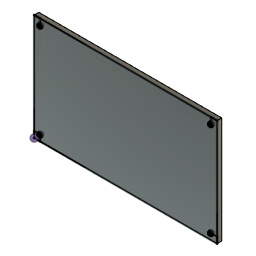
noyce 64 button backing (Autodesk Fusion 360 design; units mm, degrees)
Autodesk Fusion 360 part; units mm, degrees
note: some values were not read from the file. Set by a fixed rule: which sketch regions a step uses.
sketch "Sketch1" plane through (0, 0, 0) normal (0, 1, 0) x (1, 0, 0)
  line L0 (0, 0) -> (79, 0)
  line L1 (79, 0) -> (79, -46)
  line L2 (79, -46) -> (0, -46)
  line L3 (0, -46) -> (0, 0)
  line L4 (79, -46) -> (76.365, -46)
  line L5 (76.365, -46) -> (76.365, -43.365)
  line L6 (79, 0) -> (79, -2.635)
  line L7 (79, -2.635) -> (76.365, -2.635)
  line L8 (0, -46) -> (2.635, -46)
  line L9 (2.635, -46) -> (2.635, -43.365)
  line L10 (0, 0) -> (2.635, 0)
  line L11 (2.635, 0) -> (2.635, -2.635)
  line L12 (2.635, -2.635) -> (0, -2.635)
  line L13 (0, -2.635) -> (0, 0)
  circle A0 centre (76.365, -43.365) radius 0.8
  circle A1 centre (76.365, -2.635) radius 0.8
  circle A2 centre (2.635, -2.635) radius 0.8
  circle A3 centre (2.635, -43.365) radius 0.8
  dimension "d1" = 46
  dimension "d2" = 79
  dimension "d5" = 2.635
  dimension "d6" = 2.635
  dimension "d7" = 2.635
  dimension "d8" = 2.635
  dimension "d9" = 2.635
  dimension "d10" = 2.635
  dimension "d11" = 2.635
  dimension "d12" = 2.635
  dimension "d13" = 1.6
  dimension "d14" = 1.6
  dimension "d15" = 1.6
  dimension "d16" = 1.6
  constraint horizontal L0
  constraint vertical L1
  constraint horizontal L2
  constraint vertical L3
  constraint coincident L0.start L3.end
  constraint perpendicular L1 L4
  constraint perpendicular L2 L5
  constraint perpendicular L0 L6
  constraint perpendicular L6 L7
  constraint perpendicular L3 L8
  constraint perpendicular L2 L9
  constraint horizontal L10
  constraint vertical L11
  constraint horizontal L12
  constraint vertical L13
  constraint coincident L5.end A0.centre
  constraint coincident L7.end A1.centre
  constraint coincident L11.end L12.start
  constraint coincident L9.end A3.centre
  measures "d1" distance of L0.start L2.end
  measures "d2" distance of L0.start L0.end
  measures "d5" distance of L1.end L4.end
  measures "d6" distance of L4.end L5.end
  measures "d7" distance of L0.end L6.end
  measures "d8" distance of L6.end L7.end
  measures "d9" distance of L2.end L8.end
  measures "d10" distance of L8.end L9.end
  measures "d11" distance of L0.start L12.end
  measures "d12" distance of L0.start L10.end
  measures "d13" diameter of A0
  measures "d14" diameter of A1
  measures "d15" diameter of A2
  measures "d16" diameter of A3
extrude "Extrude2" add sketch "Sketch1" along normal blind 2 contours L0 L1 L2 L3 L4 L6 L8 L11 L12 A2 makes body 1
extrude "Extrude1" add sketch "Sketch1" along normal blind 2 separate body contours L0 L3 L10 L11 L12 L13 A2 | L0 L1 L2 L3 L4 L6 L8 L11 L12 A2 | L11 L12 A2 | L11 L12 A2 | A0 | A1 | A3 makes body 2
extrude "Extrude3" cut sketch "Sketch1" along normal blind 4 contours L11 L12 A2 | L11 L12 A2 | A0 | A1 | A3 bodies 2
